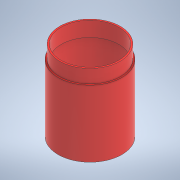
# Autodesk Inventor part: red_base
Saved by Autodesk Inventor 2021 (Build 250183000, 183)
## iProperties
Created: 2026-10-08
Part Number: red_base
Material: Generic
Document SubType Name: Modeling
Designer: alolo
Density: 1 g/cm^3
Appearance: Default
Author: alolo
Autodesk Inventor part; units mm, degrees
ref_plane "YZ Plane" through (0, 0, 0) normal (1, 0, 0) x (0, 1, 0)
ref_plane "XZ Plane" through (0, 0, 0) normal (0, 1, 0) x (-1, 0, 0)
ref_plane "XY Plane" through (0, 0, 0) normal (0, 0, 1) x (1, 0, 0)
sketch "Sketch1" plane through (0, 0, 0) normal (0, 0, 1) x (1, 0, 0)
  line L0 (0, 0) -> (31, 0)
  line L1 (31, 0) -> (31, 65)
  line L2 (31, 65) -> (29.5, 65)
  line L3 (29.5, 65) -> (29.5, 78)
  line L4 (29.5, 78) -> (28, 78)
  line L5 (28, 76.5) -> (28, 76.5)
  line L6 (28, 78) -> (28, 63.5)
  line L7 (28, 63.5) -> (29.5, 63.5)
  line L8 (29.5, 63.5) -> (29.5, 1.5)
  line L9 (29.5, 1.5) -> (0, 1.5)
  line L10 (0, 0) -> (0, 76.5) construction
  line L11 (0, 0) -> (0, 1.5)
  dimension "d1" = 31
  dimension "d2" = 65
  dimension "d3" = 1.5
  dimension "d4" = 13
  dimension "d5" = 1.5
  dimension "d6" = 1.5
  constraints: 24 end point, 4 perpendicular, 2 horizontal, 2 vertical, 1 collinear, 1 point on line, 2 other
  measures "d1" distance of L0.start L0.end
  measures "d2" distance of L0.end L1.end
  measures "d3" distance of L1.end L2.end
  measures "d4" distance of L2.end L3.end
  measures "d5" distance of L4.end L3.end
  measures "d6" distance between parallel lines of L8 L1
revolve "Revolution1" add sketch "Sketch1" angle 360 about axis through (0, 0, 0) along (0, 1, 0)
body "Solid1"
